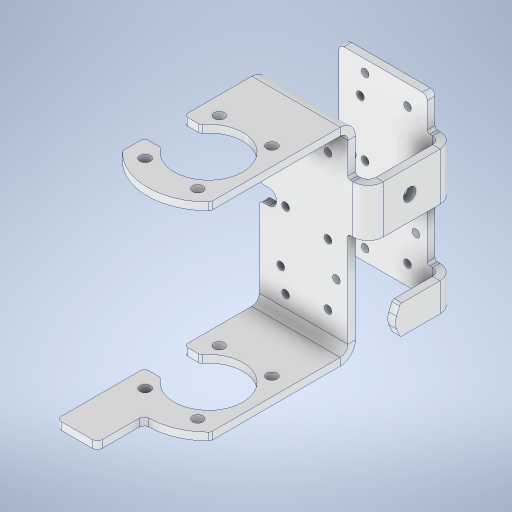
# Autodesk Inventor part: Left Gantry Guide
Saved by Autodesk Inventor 2024 (Build 280153000, 153)
## iProperties
Created: 2024-12-25
Part Number: Left Gantry Guide
Material: Aluminum 6061
Document SubType Name: Sheet Metal
Designer: Ishaan
Density: 2.7 g/cm^3
Sheet Metal Rule: SendCutSend_1-8_Alu
Appearance: Aluminum - Flat
Flat Pattern Width: 11.6413 cm
Flat Pattern Length: 23.1913 cm
Flat Pattern Area: 269.978 cm^2
Sheet Metal Width: 116.413 mm
Sheet Metal Length: 231.913 mm
Sheet Metal Area: 26997.814 mm^2
Author: Ishaan
Autodesk Inventor part; units mm, degrees
ref_plane "YZ Plane" through (0, 0, 0) normal (1, 0, 0) x (0, 1, 0)
ref_plane "XZ Plane" through (0, 0, 0) normal (0, 1, 0) x (-1, 0, 0)
ref_plane "XY Plane" through (0, 0, 0) normal (0, 0, 1) x (1, 0, 0)
sketch "Sketch1" plane through (0, 0, 0) normal (0, 0, 1) x (1, 0, 0)
  line L0 (18.5, -40.1) -> (-18.5, -40.1)
  line L1 (-18.5, -40.1) -> (-18.5, 40.1)
  line L2 (-18.5, 40.1) -> (18.5, 40.1)
  line L3 (18.5, 40.1) -> (18.5, -40.1)
  line L4 (18.5, -40.1) -> (-18.5, 40.1) construction
  line L5 (-18.5, -40.1) -> (18.5, 40.1) construction
  point P0 (0, 0)
  dimension "d0" = 37
  dimension "d1" = 80.2
extrude "Plate1" add sketch "Sketch1" along normal blind 3.175
sketch "Sketch2" plane through (18.5, -40.1, 3.175) normal (0, -1, 0) x (1, 0, 0)
  line L0 (-37, 0) -> (0, 0)
  line L1 (0, 0) -> (0, 96.825)
  line L2 (0, 96.825) -> (-37, 96.825)
  line L3 (-37, 96.825) -> (-37, 0)
  constraints: 6 end point, 1 horizontal, 1 perpendicular, 1 vertical
edge flange "Flange1" height 100 angle 90 thickness 3.175 bend radius 3.175 thickness toward (0, -1, 0) relief straight relief width 3.175 relief depth 1.5875 edges at (0, -40.1, 3.175) wall of the first edge with corners at (-18.5, -40.1, 3.175) (18.5, -40.1, 3.175) (18.5, -40.1, 100) (-18.5, -40.1, 100)
bend "Bend1"
corner "Corner1"
sketch "Sketch3" plane through (-18.5, 40.1, 3.175) normal (0, 1, 0) x (-1, 0, 0)
  line L0 (-37, 0) -> (0, 0)
  line L1 (0, 0) -> (0, 96.825)
  line L2 (0, 96.825) -> (-37, 96.825)
  line L3 (-37, 96.825) -> (-37, 0)
  constraints: 6 end point, 1 horizontal, 1 perpendicular, 1 vertical
edge flange "Flange2" height 100 angle 90 thickness 3.175 bend radius 3.175 thickness toward (0, 1, 0) relief straight relief width 3.175 relief depth 1.5875 edges at (0, 40.1, 3.175) wall of the first edge with corners at (18.5, 40.1, 3.175) (-18.5, 40.1, 3.175) (-18.5, 40.1, 100) (18.5, 40.1, 100)
bend "Bend2"
corner "Corner2"
sketch "Sketch4" plane through (-18.5, -43.275, 100) normal (0, -1, 0) x (1, 0, 0)
  line L0 (35.5, -73.9911) -> (1.5, -73.9911) construction
  line L1 (1.5, -73.9911) -> (1.5, -40.1089) construction
  line L2 (1.5, -40.1089) -> (35.5, -40.1089) construction
  line L3 (35.5, -40.1089) -> (35.5, -73.9911) construction
  line L4 (35.5, -73.9911) -> (1.5, -40.1089) construction
  line L5 (1.5, -73.9911) -> (35.5, -40.1089) construction
  circle A0 centre (18.5, -57.05) radius 24 construction
  line L6 (0, 0) -> (37, 0) construction
  circle A1 centre (18.5, -57.05) radius 25.5
  line L7 (37, -74.5999) -> (0, -74.5999)
  line L8 (0, -74.5999) -> (0, -39.5001)
  line L9 (0, -39.5001) -> (37, -39.5001)
  line L10 (37, -39.5001) -> (37, -74.5999)
  line L11 (37, -74.5999) -> (0, -39.5001) construction
  line L12 (0, -74.5999) -> (37, -39.5001) construction
  line L13 (29.5, -72.55) -> (7.5, -72.55) construction
  line L14 (7.5, -72.55) -> (7.5, -41.55) construction
  line L15 (7.5, -41.55) -> (29.5, -41.55) construction
  line L16 (29.5, -41.55) -> (29.5, -72.55) construction
  line L17 (29.5, -72.55) -> (7.5, -41.55) construction
  line L18 (7.5, -72.55) -> (29.5, -41.55) construction
  line L19 (37, -100) -> (0, -100) construction
  line L20 (0, -93.65) -> (37, -93.65) projected
  line L21 (37, 0) -> (37, -93.65) projected
  line L22 (0, 0) -> (37, 0) projected
  line L23 (0, -93.65) -> (0, 0) projected
  circle A2 centre (7.5, -41.55) radius 2 construction
  circle A3 centre (29.5, -41.55) radius 2 construction
  circle A4 centre (29.5, -72.55) radius 2 construction
  circle A5 centre (7.5, -72.55) radius 2 construction
  circle A6 centre (18.5, -57.05) radius 14.375
  line L24 (18.5, -57.05) -> (0, -57.05) construction
  line L25 (18.5, -48.8) -> (0, -48.8)
  line L26 (0, -65.3) -> (18.5, -65.3)
  arc A7 (18.5, -65.3) -> (18.5, -48.8) centre (18.5, -57.05) ccw
  arc A8 (0, -48.8) -> (0, -65.3) centre (0, -57.05) ccw
  line L27 (40, -70.7613) -> (40, -43.3387)
  point P0 (18.5, -100)
  point P1 (18.5, 0)
  point P2 (9.25, -57.05)
  point P3 (0, -39.5001)
  point P4 (37, -39.5001)
  point P5 (0, -65.3)
  point P6 (6.7281, -65.3)
  point P7 (6.7281, -48.8)
  point P8 (0, -48.8)
  point P9 (37, -74.5999)
  dimension "d25" = 48
  dimension "d23" = 34
  dimension "d26" = 1.5
  dimension "d28" = 1.5
  dimension "d29" = 22
  dimension "d30" = 31
  dimension "d31" = 42.95
  dimension "d32" = 4
  dimension "d33" = 28.75
  dimension "d34" = 16.5
  dimension "d46" = 3
  constraints: 46 end point, 11 coincident, 8 centre point, 8 midpoint, 7 parallel, 7 point on circle, 4 perpendicular, 4 tangent, 3 equal radius, 3 horizontal, 1 point on line, 1 vertical, 1 vertical alignment, 3 other
  measures "d23" distance of L1.end L2.end
  measures "d26" distance between parallel lines of L8 L1
  measures "d29" distance of L14.end L15.end
  measures "d30" distance of L13.end L14.end
  measures "d31" distance from line of point (18.5, -57.05) L19
  measures "d32" diameter of A2
  measures "d33" diameter of A6
  measures "d34" diameter of A8
  measures "d46" distance between parallel lines of L10 L27
extrude "Extrusion1" cut sketch "Sketch4" against normal up to surface (3.175 mm away) contours A1 L23 L22 L21 | L25 A6 L26 L8 | L25 A7 L26 A6 | A6 L26 A7 L25
hole "Hole1" at (-11, -43.275, 27.45) at (-11, -43.275, 58.45) at (11, -43.275, 58.45) at (11, -43.275, 27.45) direction (0, 1, 0) diameter 4.4 depth 3.175
mirror "Mirror1" about plane through (0, 0, 0) normal (0, 1, 0) of "Extrusion1", "Hole1"
sketch "Sketch5" plane through (0, 0, 3.175) normal (0, 0, 1) x (1, 0, 0)
  line L0 (10.236, -3) -> (10.236, -28.472) construction
  line L1 (18.5, 36.925) -> (18.5, -36.925) projected
  line L2 (10.236, -15.736) -> (13.736, -15.736) construction
  line L3 (18.5, -40.1) -> (-18.5, -40.1) projected
  circle A0 centre (10.236, -3) radius 6 construction
  circle A1 centre (10.236, -28.472) radius 6 construction
  circle A2 centre (13.736, -15.736) radius 6.736 construction
  line L4 (10.236, -22.472) -> (35.0958, -22.472) construction
  line L5 (10.236, -9) -> (35.0958, -9) construction
  line L6 (18.5, 23) -> (53.1345, 23) construction
  line L7 (53.1345, 23) -> (53.1345, 3) construction
  line L8 (53.1345, 3) -> (18.5, 3) construction
  line L9 (18.5, 3) -> (18.5, 23) construction
  line L10 (18.5, 23) -> (20.65, 23)
  line L11 (20.65, 23) -> (20.65, 3)
  line L12 (20.65, 3) -> (18.5, 3)
  line L13 (18.5, 3) -> (18.5, 23)
  line L14 (27, 23) -> (27, 3) construction
  line L15 (10.236, 28.472) -> (10.236, -28.472) construction
  point P0 (0, 0)
  point P1 (18.5, 13)
  point P2 (18.5, 23)
  point P3 (18.5, 3)
  point P4 (10.236, 0)
  dimension "d52" = 12
  dimension "d49" = 3.5
  dimension "d51" = 8.264
  dimension "d53" = 13.472
  dimension "d61" = 20
  dimension "d62" = 22
  dimension "d127" = 6.35
  dimension "d128" = 27
  dimension "d145" = 3
  constraints: 28 end point, 6 coincident, 6 horizontal, 4 parallel, 4 perpendicular, 4 point on line, 3 midpoint, 2 collinear, 2 vertical alignment, 1 centre point, 1 horizontal alignment, 1 tangent, 1 vertical, 4 other
  measures "d49" distance of L2.start L2.end
  measures "d51" distance from line of L1 L0.end
  measures "d53" diameter of A2
  measures "d61" distance of L8.end L6.start
  measures "d62" distance from line of point (18.5, 13) L5
  measures "d127" distance between parallel lines of L11 L14
  measures "d128" distance from line of L14 point (0, 0)
  measures "d145" vertical distance of L0.start point (0, 0)
hole "Hole2" at (10.236, -3, 3.175) at (10.236, -28.472, 3.175) at (13.736, -15.736, 3.175) at (10.236, 28.472, 3.175) direction (0, 0, -1) diameter 3.2 end through all
extrude "Extrusion3" add sketch "Sketch5" against normal up to surface (3.175 mm away)
sketch "Sketch6" plane through (23.825, 3, -3.175) normal (1, 0, 0) x (0, 1, 0)
  line L0 (20, 0) -> (0, 0)
  line L1 (0, 0) -> (0, -26.925)
  line L2 (0, -26.925) -> (20, -26.925)
  line L3 (20, -26.925) -> (20, 0)
  constraints: 6 end point, 1 horizontal, 1 perpendicular, 1 vertical
edge flange "Flange3" height 30.1 angle 90 thickness 3.175 bend radius 3.175 thickness toward (1, 0, 0) relief straight relief width 3.175 relief depth 1.5875 edges at (20.65, 13, 0) wall of the first edge with corners at (23.825, 23, -3.175) (23.825, 3, -3.175) (23.825, 3, -30.1) (23.825, 23, -30.1)
bend "Bend3"
corner "Corner3"
sketch "Sketch7" plane through (23.825, 3, -30.1) normal (0, 0, -1) x (-1, 0, 0)
  line L0 (0, 20) -> (0, 0)
  line L1 (0, 0) -> (5.325, 0)
  line L2 (5.325, 0) -> (5.325, 20)
  line L3 (5.325, 20) -> (0, 20)
  constraints: 6 end point, 1 horizontal, 1 perpendicular, 1 vertical
edge flange "Flange4" height 3 angle 90 thickness 3.175 bend radius 3.175 thickness toward (0, 0, -1) relief straight relief width 3.175 relief depth 1.5875 edges at (23.825, 13, -30.1) wall of the first edge with corners at (23.825, 23, -30.1) (23.825, 3, -30.1) (18.5, 3, -30.1) (18.5, 23, -30.1)
bend "Bend4"
corner "Corner4"
sketch "Sketch8" plane through (18.5, 3, -33.275) normal (0, 0, -1) x (-1, 0, 0)
  circle A0 centre (4.764, -18.736) radius 1.6 projected
  circle A1 centre (8.264, -31.472) radius 1.6 projected
  circle A2 centre (8.264, -6) radius 1.6 projected
  line L0 (37, 33.925) -> (0, 33.925) projected
  line L1 (0, 20) -> (0, 33.925) projected
  line L2 (0, 20) -> (-2.15, 20) projected
  line L3 (-2.15, 20) -> (-2.15, 0) projected
  line L4 (-2.15, 0) -> (0, 0) projected
  line L5 (0, -39.925) -> (0, 0) projected
  line L6 (0, -39.925) -> (37, -39.925) projected
  line L7 (37, 33.925) -> (37, -39.925) projected
  line L8 (0, 20) -> (0, 0) projected
  line L9 (0, 20) -> (37, 20)
  line L10 (0, -39.925) -> (0, 0) projected
  line L11 (0, -39.736) -> (37, -39.736)
  circle A3 centre (8.264, -31.472) radius 8.264
  circle A4 centre (8.264, 25.472) radius 1.6 projected
  circle A5 centre (8.264, 25.472) radius 8.264
  line L12 (0, 33.736) -> (37, 33.736)
  point P0 (18.5, -3)
  point P1 (0, -39.736)
  point P2 (6.7536, 20)
  point P3 (9.7744, 20)
  constraints: 6 end point, 5 point on line, 4 tangent, 3 perpendicular, 2 centre point, 2 coincident
extrude "Extrusion4" add sketch "Sketch8" against normal up to surface (3.175 mm away) contours L7 L9 A5 L12 | L12 A5 L1 | L7 L11 A3 L5 L8 L9 A5 | A5 L9 | A5 L9 L1 | A5 L9 | L11 L5 A3 | A3
sketch "Sketch9" plane through (27, 3, -3.175) normal (1, 0, 0) x (0, 0, -1)
  line L0 (23.75, 0) -> (23.75, 20) projected
  line L1 (0, 20) -> (23.75, 20) projected
  line L2 (0, 20) -> (0, 0) projected
  line L3 (23.75, 0) -> (0, 0) projected
  line L4 (23.75, 20) -> (0, 20) construction
  line L5 (0, 20) -> (0, 0) construction
  line L6 (0, 0) -> (23.75, 0) construction
  line L7 (23.75, 0) -> (23.75, 20) construction
  line L8 (23.75, 20) -> (0, 0) construction
  line L9 (0, 20) -> (23.75, 0) construction
  point P0 (-3.175, -3)
  point P1 (11.875, 10)
  point P2 (11.875, 10)
  point P3 (11.025, 10)
  dimension "d144" = 0.85
  constraints: 12 end point, 2 midpoint, 2 parallel, 1 coincident, 1 horizontal, 1 horizontal alignment, 1 perpendicular
  measures "d144" distance of point (11.025, 10) point (11.875, 10)
hole "Hole3" at (27, 13, -14.2) direction (-1, 0, 0) diameter 5.3 end through all
sketch "Sketch10" plane through (20.65, 3, -30.1) normal (0, 0, 1) x (1, 0, 0)
  line L0 (5.4993, 20) -> (5.4993, 0) projected
  line L1 (5.4993, 0) -> (0, 0) projected
  line L2 (0, 20) -> (0, 0) projected
  line L3 (-2.15, 20) -> (0, 20) projected
  line L4 (0, 0) -> (-2.15, 0) projected
  line L5 (0, 20) -> (5.4993, 20) projected
  circle A0 centre (-10.414, -6) radius 9 construction
  circle A1 centre (-6.914, -18.736) radius 9 construction
  circle A2 centre (-10.414, -31.472) radius 9 construction
  line L6 (-2.15, 33.736) -> (-2.15, 20) projected
  circle A3 centre (-10.414, -6) radius 1.6 projected
  circle A4 centre (-6.914, -18.736) radius 1.6 projected
  circle A5 centre (-10.414, -31.472) radius 1.6 projected
  line L7 (-39.15, 33.736) -> (-2.15, 33.736) projected
  line L8 (-39.15, -39.736) -> (-39.15, 33.736) projected
  line L9 (-2.15, -39.736) -> (-39.15, -39.736) projected
  line L10 (-2.15, 0) -> (-2.15, -39.736) projected
  line L11 (-28.15, 28.736) -> (-28.15, -34.736) construction
  line L12 (-30.15, 19.5) -> (-30.15, -25.5) construction
  circle A6 centre (-10.414, 25.472) radius 1.6 projected
  point P0 (-20.65, -3)
  point P1 (-10.414, -31.472)
  point P2 (-10.414, -6)
  point P3 (-6.914, -18.736)
  point P4 (-28.15, -3)
  point P5 (-39.15, -3)
  point P6 (-28.15, -3)
  point P7 (-30.15, -3)
  dimension "d129" = 18
  dimension "d150" = 5
  dimension "d151" = 11
  dimension "d152" = 45
  dimension "d153" = 9
  constraints: 8 coincident, 4 end point, 3 centre point, 3 midpoint, 2 equal radius, 2 horizontal alignment, 2 vertical
  measures "d129" diameter of A0
  measures "d150" distance from line of L9 L11.end
  measures "d151" distance between parallel lines of L8 L11
  measures "d152" distance of L12.start L12.end
  measures "d153" distance between parallel lines of L8 L12
hole "Hole4" at (-7.5, 31.736, -30.1) at (-7.5, 0, -30.1) at (-7.5, -31.736, -30.1) direction (0, 0, -1) diameter 3.2 end through all both
hole "Hole5" at (-9.5, 22.5, -30.1) at (-9.5, -22.5, -30.1) direction (0, 0, -1) diameter 3.2 end through all both
sketch "Sketch13" plane through (20.65, 3, -33.275) normal (0, 0, -1) x (-1, 0, 0)
  circle A0 centre (30.15, -25.5) radius 1.6 projected
  circle A1 centre (30.15, 19.5) radius 1.6 projected
  circle A2 centre (28.15, -34.736) radius 1.6 projected
  circle A3 centre (28.15, -3) radius 1.6 projected
  circle A4 centre (28.15, 28.736) radius 1.6 projected
  circle A5 centre (10.414, -6) radius 1.6 projected
  circle A6 centre (6.914, -18.736) radius 1.6 projected
  circle A7 centre (10.414, -31.472) radius 1.6 projected
  circle A8 centre (10.414, 25.472) radius 1.6 projected
  line L0 (0, 20) -> (0, 0) projected
  line L1 (2.15, 0) -> (0, 0) projected
  line L2 (2.15, 0) -> (2.15, -39.736) projected
  line L3 (2.15, -39.736) -> (39.15, -39.736) projected
  line L4 (39.15, -39.736) -> (39.15, 33.736) projected
  line L5 (39.15, 33.736) -> (2.15, 33.736) projected
  line L6 (2.15, 33.736) -> (2.15, 20) projected
  line L7 (0, 20) -> (2.15, 20) projected
  line L8 (2.15, -39.736) -> (0, -39.736)
  line L9 (0, -39.736) -> (0, -27.736)
  line L10 (0, -27.736) -> (2.15, -27.736)
  line L11 (2.15, -27.736) -> (2.15, -39.736)
  line L12 (0, 20) -> (0, 0) projected
  point P0 (20.65, -3)
  point P1 (2.15, -27.736)
  dimension "d154" = 12
  constraints: 8 end point, 2 parallel, 1 collinear, 1 horizontal, 1 perpendicular
  measures "d154" distance of L8.end L9.end
extrude "Extrusion7" add sketch "Sketch13" against normal up to surface (3.175 mm away) contours L2 L8 L9 L10
sketch "Sketch14" plane through (23.825, -24.736, -26.925) normal (1, 0, 0) x (0, 1, 0)
  line L0 (-12, 0) -> (0, 0)
  line L1 (0, 0) -> (0, 33.65)
  line L2 (0, 33.65) -> (-12, 33.65)
  line L3 (-12, 33.65) -> (-12, 0)
  constraints: 6 end point, 1 horizontal, 1 perpendicular, 1 vertical
edge flange "Flange5" height 40 angle 90 thickness 3.175 bend radius 3.175 thickness toward (1, 0, 0) relief straight relief width 3.175 relief depth 1.5875 edges at (20.65, -30.736, -30.1) wall of the first edge with corners at (23.825, -36.736, -26.925) (23.825, -24.736, -26.925) (23.825, -24.736, 6.725) (23.825, -36.736, 6.725)
bend "Bend5"
corner "Corner5"
sketch "Sketch15" plane through (27, -36.736, 6.725) normal (1, 0, 0) x (0, 0, -1)
  circle A0 centre (20.925, 49.736) radius 2.65 construction
  line L0 (33.65, 0) -> (33.65, 12) projected
  line L1 (0, 12) -> (33.65, 12) projected
  line L2 (0, 0) -> (0, 12) projected
  line L3 (33.65, 0) -> (0, 0) projected
  circle A1 centre (20.925, 6) radius 6
  line L4 (0, 12) -> (33.65, 12) projected
  line L5 (33.65, 0) -> (0, 0) projected
  line L6 (16.9159, 0) -> (15.3817, 3.7039)
  line L7 (15.3817, 8.2961) -> (16.9159, 12)
  point P0 (6.725, 36.736)
  point P1 (16.9159, 0)
  point P2 (16.9159, 12)
  dimension "d167" = 135
  constraints: 4 end point, 4 tangent, 2 point on circle, 2 point on line, 2 vertical alignment, 1 centre point
  measures "d167" angle of L6 L7
extrude "Extrusion8" cut sketch "Sketch15" against normal up to surface (3.175 mm away) contours L3 L2 L1 L7 A1 L6
fillet "Fillet1" radius 1 5 edges at (18.5, 3, 1.5875) (18.5, 23, 1.5875) (18.5, 23, -31.6875) (18.5, 3, -31.6875) (18.5, -24.736, -31.6875)
fillet "Fillet2" radius 2 3 edges at (-18.5, -36.736, -31.6875) (18.5, 36.736, -31.6875) (-18.5, 36.736, -31.6875)
fillet "Fillet3" radius 1.5 12 edges at (18.5, -41.6875, 60.4999) (-18.5, -41.6875, 60.4999) (-11.7719, -41.6875, 34.7) (-11.7719, -41.6875, 51.2) (-18.5, -41.6875, 51.2) (-18.5, -41.6875, 34.7) (18.5, 41.6875, 60.4999) (-11.7719, 41.6875, 34.7) (-18.5, 41.6875, 34.7) (-11.7719, 41.6875, 51.2) (-18.5, 41.6875, 51.2) (-18.5, 41.6875, 60.4999)
fillet "Fillet6" radius 1 2 edges at (25.4125, -24.736, -10.1909) (25.4125, -36.736, -10.1909)
sketch "Sketch11" plane through (20.65, 3, -33.275) normal (0, 0, -1) x (-1, 0, 0)
  line L0 (0, 20) -> (1.15, 20) projected
  line L1 (0, 20) -> (0, 0) projected
  line L2 (1.15, 0) -> (0, 0) projected
  line L3 (39.15, -3) -> (35.15, -3) construction
  line L4 (39.15, 0.25) -> (35.15, 0.25)
  line L5 (35.15, -6.25) -> (39.15, -6.25)
  arc A0 (39.15, -6.25) -> (39.15, 0.25) centre (39.15, -3) ccw
  arc A1 (35.15, 0.25) -> (35.15, -6.25) centre (35.15, -3) ccw
  arc A2 (39.15, 31.736) -> (37.15, 33.736) centre (37.15, 31.736) ccw projected
  line L6 (37.15, 33.736) -> (4.15, 33.736) projected
  arc A3 (4.15, 33.736) -> (2.15, 31.736) centre (4.15, 31.736) ccw projected
  line L7 (2.15, 31.736) -> (2.15, 21) projected
  arc A4 (1.15, 20) -> (2.15, 21) centre (1.15, 21) ccw projected
  arc A5 (2.15, -1) -> (1.15, 0) centre (1.15, -1) ccw projected
  line L8 (2.15, -1) -> (2.15, -26.736) projected
  line L9 (0, -39.736) -> (37.15, -39.736) projected
  arc A6 (37.15, -39.736) -> (39.15, -37.736) centre (37.15, -37.736) ccw projected
  line L10 (39.15, -37.736) -> (39.15, 31.736) projected
  circle A7 centre (28.15, -3) radius 1.6 projected
  line L11 (39.15, -37.736) -> (39.15, 31.736) projected
  arc A8 (1.15, -27.736) -> (2.15, -26.736) centre (1.15, -26.736) ccw projected
  line L12 (1.15, -27.736) -> (0, -27.736) projected
  line L13 (0, -27.736) -> (0, -39.736) projected
  point P0 (20.65, -3)
  point P1 (37.15, -3)
  dimension "d130" = 6.5
  dimension "d131" = 4
  constraints: 8 end point, 4 point on circle, 4 tangent, 2 centre point, 2 midpoint, 1 parallel, 1 perpendicular, 1 point on line
  measures "d130" diameter of A1
  measures "d131" distance of L3.start L3.end
extrude "Extrusion5" cut sketch "Sketch11" against normal up to surface (36.45 mm away) contours L10 L5 A1 L4 | A0 L10
fillet "Fillet4" radius 1.5 4 edges at (-18.5, 3.25, 1.5875) (-18.5, -3.25, 1.5875) (-18.5, -3.25, -31.6875) (-18.5, 3.25, -31.6875)
ref_plane "Work Plane1" through (0, 0, -15.05) normal (0, 0, -1) x (-1, 0, 0)
ref_plane "Work Plane2" through (0, 0, -7.55) normal (0, 0, -1) x (-1, 0, 0)
ref_plane "Work Plane3" through (0, 0, -22.55) normal (0, 0, -1) x (-1, 0, 0)
ref_plane "Work Plane4" through (0, 0, -15.05) normal (0, 0, -1) x (-1, 0, 0)
sketch "Sketch12" plane through (-18.5, -43.275, 6.35) normal (0, -1, 0) x (1, 0, 0)
  arc A0 (1.5, 28.35) -> (0, 26.85) centre (1.5, 26.85) ccw projected
  line L0 (0, 0) -> (0, 26.85) projected
  line L1 (0, 0) -> (37, 0) projected
  line L2 (37, 53.5411) -> (37, 0) projected
  arc A1 (37, 53.5411) -> (36.5625, 54.5999) centre (35.5, 53.5411) ccw projected
  arc A2 (36.5625, 54.5999) -> (0.4375, 54.5999) centre (18.5, 36.6) ccw projected
  arc A3 (0.4375, 54.5999) -> (0, 53.5411) centre (1.5, 53.5411) ccw projected
  line L3 (0, 46.35) -> (0, 53.5411) projected
  arc A4 (0, 46.35) -> (1.5, 44.85) centre (1.5, 46.35) ccw projected
  line L4 (1.5, 44.85) -> (5.9719, 44.85) projected
  arc A5 (5.9719, 44.85) -> (7.1557, 45.4287) centre (5.9719, 46.35) ccw projected
  arc A6 (7.1557, 27.7713) -> (7.1557, 45.4287) centre (18.5, 36.6) ccw projected
  arc A7 (7.1557, 27.7713) -> (5.9719, 28.35) centre (5.9719, 26.85) ccw projected
  line L5 (5.9719, 28.35) -> (1.5, 28.35) projected
  circle A8 centre (29.5, 21.1) radius 2.2 projected
  circle A9 centre (29.5, 52.1) radius 2.2 projected
  circle A10 centre (7.5, 52.1) radius 2.2 projected
  circle A11 centre (7.5, 21.1) radius 2.2 projected
  line L6 (0, 53.5411) -> (0, 81.6)
  line L7 (0, 81.6) -> (17, 81.6)
  line L8 (17, 81.6) -> (17, 62.1)
  line L9 (17, 62.1) -> (18.5, 62.1)
  arc A12 (36.5625, 54.5999) -> (0.4375, 54.5999) centre (18.5, 36.6) ccw projected
  point P0 (18.5, -6.35)
  dimension "d137" = 18.5
  dimension "d138" = 1.5
  dimension "d139" = 45
  constraints: 8 end point, 2 perpendicular, 1 point on circle, 1 tangent, 1 vertical
  measures "d137" distance from line of L6 A2.centre
  measures "d138" distance from line of L8 A6.centre
  measures "d139" distance from line of A2.centre L7
extrude "Extrusion6" add sketch "Sketch12" against normal up to surface (3.175 mm away) contours A2 A3 L6 L7 L8 L9
fillet "Fillet5" radius 2 3 edges at (-1.5, -41.6875, 68.45) (-1.5, -41.6875, 87.95) (-18.5, -41.6875, 87.95)
equation "\"d28\" = d26"
equation "\"d44\" = Thickness"
equation "\"d111\" = Thickness"
equation "\"d2\" = Thickness"
equation "\"d3\" = BendReliefWidth"
equation "\"d4\" = BendReliefDepth"
equation "\"d5\" = MinimumRemnant"
equation "\"d6\" = TransitionRadius"
equation "\"d9\" = BendRadius"
equation "\"d10\" = CornerReliefSize"
equation "\"d11\" = GapSize"
equation "\"d12\" = JacobiRadiusSize"
equation "\"d13\" = BendReliefWidth"
equation "\"d14\" = BendReliefDepth"
equation "\"d15\" = MinimumRemnant"
equation "\"d16\" = TransitionRadius"
equation "\"d19\" = BendRadius"
equation "\"d20\" = CornerReliefSize"
equation "\"d21\" = GapSize"
equation "\"d22\" = JacobiRadiusSize"
equation "\"d66\" = BendReliefWidth"
equation "\"d67\" = BendReliefDepth"
equation "\"d68\" = MinimumRemnant"
equation "\"d69\" = TransitionRadius"
equation "\"d72\" = BendRadius"
equation "\"d73\" = CornerReliefSize"
equation "\"d74\" = GapSize"
equation "\"d75\" = JacobiRadiusSize"
equation "\"d76\" = BendReliefWidth"
equation "\"d77\" = BendReliefDepth"
equation "\"d78\" = MinimumRemnant"
equation "\"d79\" = TransitionRadius"
equation "\"d82\" = BendRadius"
equation "\"d84\" = CornerReliefSize"
equation "\"d85\" = GapSize"
equation "\"d86\" = JacobiRadiusSize"
equation "\"BendReliefWidth\" = Thickness"
equation "\"BendReliefDepth\" = 0.5 * Thickness"
equation "\"CornerReliefSize\" = 4 * Thickness"
equation "\"MinimumRemnant\" = 2 * Thickness"
equation "\"TransitionRadius\" = BendRadius"
equation "\"JacobiRadiusSize\" = BendRadius"
equation "\"GapSize\" = Thickness"
equation "\"Thickness\" = 3.175"
equation "\"BendRadius\" = 3.175"
body "Solid1"
